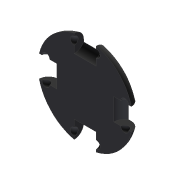
# Autodesk Inventor part: omni_wheel_cover_in
Saved by Autodesk Inventor 2017 (Build 210142000, 142)
## iProperties
Created: 2018-10-27
Part Number: omni_wheel_cover_in
Material: Generic
Document SubType Name: Modeling
Designer: mfans
Density: 1 g/cm^3
Appearance: Default
Author: mfans
Autodesk Inventor part; units mm, degrees
ref_plane "YZ Plane" through (0, 0, 0) normal (1, 0, 0) x (0, 1, 0)
ref_plane "XZ Plane" through (0, 0, 0) normal (0, 1, 0) x (-1, 0, 0)
ref_plane "XY Plane" through (0, 0, 0) normal (0, 0, 1) x (1, 0, 0)
sketch "Sketch1" plane through (0, 0, 0) normal (0, 1, 0) x (-1, 0, 0)
  circle A0 centre (0, 0) radius 30
  dimension "d0" = 60
  constraints: 1 centre point, 1 coincident
  measures "d0" diameter of A0
extrude "Extrusion1" add sketch "Sketch1" along normal blind 6
fillet "Fillet1" radius 6 1 edges at (30, 6, 0)
sketch "Sketch2" plane through (0, 0, 0) normal (0, -1, 0) x (1, 0, 0)
  line L0 (-7, -25) -> (7, -25)
  line L1 (7, -25) -> (7, -18)
  line L2 (7, -18) -> (-7, -18)
  line L3 (-7, -18) -> (-7, -25)
  line L4 (-7, -25) -> (7, -18) construction
  line L5 (7, -25) -> (-7, -18) construction
  arc A0 (-4.5, -25) -> (-9.5, -25) centre (-7, -25) ccw
  arc A1 (9.5, -25) -> (4.5, -25) centre (7, -25) ccw
  line L6 (-9.5, -25) -> (9.5, -25)
  point P0 (0, 0)
  point P1 (0, -21.5)
  dimension "d4" = 14
  dimension "d5" = 7
  dimension "d6" = 18
  dimension "d7" = 5
  dimension "d8" = 5
  constraints: 14 end point, 4 point on circle, 2 centre point, 2 coincident, 2 horizontal, 2 midpoint, 2 parallel, 2 point on line, 1 perpendicular
  measures "d4" distance of L2.end L1.end
  measures "d5" distance of L0.end L1.end
  measures "d6" distance from line of point (0, 0) L2
  measures "d7" diameter of A0
  measures "d8" diameter of A1
revolve "Revolution1" cut sketch "Sketch2" angle 360 about axis through (-7, 0, -25) along (1, 0, 0)
pattern_circular "Circular Pattern1" count 4 over 360 about axis through (0, -10, 0) along (0, 1, 0) of "Revolution1"
body "Solid1"
